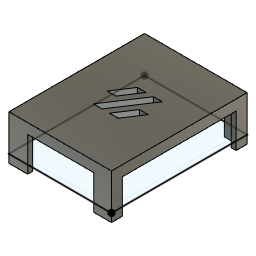
BME Box v3 (Autodesk Fusion 360 design; units mm, degrees)
Autodesk Fusion 360 part; units mm, degrees
sketch "Sketch1" plane through (0, 0, 0) normal (0, 0, 1) x (1, 0, 0)
  line L0 (0, 0) -> (31, 0)
  line L1 (31, 0) -> (31, 41)
  line L2 (31, 41) -> (0, 41)
  line L3 (0, 41) -> (0, 0)
  line L4 (1.5, 39.5) -> (29.5, 39.5)
  line L5 (29.5, 39.5) -> (29.5, 1.5)
  line L6 (29.5, 1.5) -> (1.5, 1.5)
  line L7 (1.5, 1.5) -> (1.5, 39.5)
  line L8 (1.5, 39.5) -> (29.5, 1.5) construction
  line L9 (29.5, 39.5) -> (1.5, 1.5) construction
  circle A0 centre (15.5, 28.7333) radius 7.5
  point P0 (15.5, 20.5)
  dimension "d1" = 31
  dimension "d2" = 41
  dimension "d3" = 28
  dimension "d4" = 38
  dimension "d5" = 15
  constraint horizontal L0
  constraint vertical L1
  constraint horizontal L2
  constraint vertical L3
  constraint coincident L0.start L3.end
  constraint horizontal L4
  constraint perpendicular L4 L5
  constraint parallel L4 L6
  constraint parallel L5 L7
  constraint coincident L8 P0
  constraint coincident L9 P0
  measures "d1" distance of L0.start L0.end
  measures "d2" distance of L0.start L2.end
  measures "d3" distance of L5.end L6.end
  measures "d4" distance of L4.end L5.end
  measures "d5" diameter of A0
extrude "Extrude1" add sketch "Sketch1" along normal blind 2 contours L0 L1 L2 L3 | L4 L5 L6 L7 makes body 1
extrude "Extrude2" add sketch "Sketch1" along normal blind 4 contours L4 L5 L6 L7 bodies 1
sketch "Sketch1 (2)" plane through (0, 0, 2) normal (0, 0, 1) x (-1, 0, 0) in component "Top"
  line L0 (-1.5, -1.5) -> (-1.5, -39.5)
  line L1 (-1.5, -39.5) -> (-29.5, -39.5)
  line L2 (-29.5, -39.5) -> (-29.5, -1.5)
  line L3 (-29.5, -1.5) -> (-1.5, -1.5)
  line L4 (0, -41) -> (0, 0)
  line L5 (0, 0) -> (-31, 0)
  line L6 (-31, 0) -> (-31, -41)
  line L7 (-31, -41) -> (0, -41)
  line L8 (0, -41) -> (-31, -41)
  line L9 (-31, -41) -> (-31, 0)
  line L10 (-31, 0) -> (0, 0)
  line L11 (0, 0) -> (0, -41)
  constraint horizontal L8
  constraint vertical L9
  constraint horizontal L10
  constraint vertical L11
  constraint coincident L5.end L6.start
  constraint coincident L4.start L7.end
extrude "Extrude1'" add sketch "Sketch1 (2)" along normal blind 10 separate body contours L0 L1 L2 L3 | L4 L5 L6 L7 L8 L9 L10 L11 makes body 2 in component "Top"
shell "Shell1" thickness 1.5 removed faces 1 at (10.3333, 27.3333, 2) on bodies 2 in component "Top"
ref_plane "WorkPlane1" through (15.5, 20.5, 12) normal (0, 0, 1) x (1, 0, 0)
sketch "Sketch2" plane through (15.5, 20.5, 12) normal (0, 0, 1) x (1, 0, 0) in component "Top"
  line L0 (0.1136, 9.8824) -> (-8.6176, 4.8413)
  line L1 (-8.6176, 4.8413) -> (-8.6176, -5.2393)
  line L2 (-8.6176, -5.2393) -> (0.1136, -10.2796)
  line L3 (0.1136, -10.2796) -> (8.8449, -5.2393)
  line L4 (8.8449, -5.2393) -> (8.8449, 4.8413)
  line L5 (8.8449, 4.8413) -> (0.1136, 9.8824)
  line L6 (-2.4502, 5.2787) -> (0.1835, 5.2787)
  line L7 (0.1835, 5.2787) -> (-3.4193, -0.2014)
  line L8 (-3.4193, -0.2014) -> (-6.053, -0.2014)
  line L9 (-6.053, -0.2014) -> (-2.4502, 5.2787)
  line L10 (-4.8021, -5.6751) -> (2.4028, 5.2866)
  line L11 (2.4028, 5.2866) -> (5.0365, 5.2866)
  line L12 (5.0365, 5.2866) -> (-2.1692, -5.6751)
  line L13 (-2.1692, -5.6751) -> (-4.8021, -5.6751)
  line L14 (2.6854, -5.6751) -> (0.0517, -5.6751)
  line L15 (0.0517, -5.6751) -> (3.6538, -0.195)
  line L16 (3.6538, -0.195) -> (6.2874, -0.195)
  line L17 (6.2874, -0.195) -> (2.6854, -5.6751)
extrude "Extrude2'" cut sketch "Sketch2" against normal blind 0.5 bodies 2 in component "Top"
extrude "Extrude3" cut 3 faces at (19.7089, 18.4783, 12) (17.2567, 22.1327, 12) (13.6047, 23.952, 12) along direction (0, 0, -1) blind 2 on bodies 2 bodies 2 in component "Top"
sketch "Sketch2 (1)" plane through (0, 41, 0) normal (0, 1, 0) x (-1, 0, 0) in component "Top"
  line L0 (-31, 2) -> (0, 2)
  line L1 (0, 2) -> (0, 12)
  line L2 (0, 12) -> (-31, 12)
  line L3 (-31, 12) -> (-31, 2)
  line L4 (-28.0584, 2) -> (-2.1668, 2)
  line L5 (-2.1668, 2) -> (-2.1668, 9.9165)
  line L6 (-2.1668, 9.9165) -> (-28.0584, 9.9165)
  line L7 (-28.0584, 9.9165) -> (-28.0584, 2)
  point P0 (-15.5, 7)
  constraint horizontal L4
  constraint vertical L5
  constraint horizontal L6
  constraint vertical L7
  constraint coincident L0 L4.start
sketch "Sketch3" plane through (31, 0, 0) normal (1, 0, 0) x (0, 1, 0) in component "Top"
  line L0 (0, 2) -> (41, 2)
  line L1 (41, 2) -> (41, 12)
  line L2 (41, 12) -> (0, 12)
  line L3 (0, 12) -> (0, 2)
  line L4 (3.2975, 9.8315) -> (37.7025, 9.8315)
  line L5 (37.7025, 9.8315) -> (37.7025, 4.1685)
  line L6 (37.7025, 4.1685) -> (3.2975, 4.1685)
  line L7 (3.2975, 4.1685) -> (3.2975, 9.8315)
  line L8 (3.2975, 9.8315) -> (37.7025, 4.1685) construction
  line L9 (37.7025, 9.8315) -> (3.2975, 4.1685) construction
  point P0 (20.5, 7)
  constraint horizontal L4
  constraint perpendicular L4 L5
  constraint parallel L4 L6
  constraint parallel L5 L7
  constraint coincident L8 P0
  constraint coincident L9 P0
extrude "Extrude5" cut sketch "Sketch3" against normal blind 35 contours L4 L5 L6 L7 bodies 2 in component "Top"
extrude "Extrude6" add 1 faces at (15.5379, 37.4608, 12) along direction (0, 0, 1) blind 1 on bodies 2 bodies 2 in component "Top"
extrude "Extrude7" add 1 faces at (9.7931, 23.8062, 11.5) along direction (0, 0, 1) blind 1.5 on bodies 2 bodies 2 in component "Top"
extrude "Extrude8" cut 1 faces at (15.5612, 35.9262, 13) along direction (0, 0, 1) blind 1 on bodies 2 bodies 2 in component "Top"
extrude "Extrude9" add sketch "Sketch1 (2)" against normal blind 2.5 bodies 2 in component "Top"
sketch "Sketch4" plane through (0, 0, 0) normal (-1, 0, 0) x (0, -1, 0) in component "Top"
  line L0 (-37.7025, 4.1685) -> (-37.7025, 9.8315)
  line L1 (-37.7025, 9.8315) -> (-3.2975, 9.8315)
  line L2 (-3.2975, 9.8315) -> (-3.2975, 4.1685)
  line L3 (-3.2975, 4.1685) -> (-37.7025, 4.1685)
  line L4 (0, -0.5) -> (0, 13)
  line L5 (0, 13) -> (-41, 13)
  line L6 (-41, 13) -> (-41, -0.5)
  line L7 (-41, -0.5) -> (0, -0.5)
  line L8 (-37.7025, 9.8315) -> (-3.2975, 9.8315)
  line L9 (-3.2975, 9.8315) -> (-3.2975, -1.832)
  line L10 (-3.2975, -1.832) -> (-37.7025, -1.832)
  line L11 (-37.7025, -1.832) -> (-37.7025, 9.8315)
  constraint horizontal L8
  constraint vertical L9
  constraint horizontal L10
  constraint vertical L11
  constraint coincident L2 L9.end
  constraint coincident L0.end L1.start
extrude "Extrude10" cut sketch "Sketch4" against normal blind 45.044 contours L0 L1 L2 L3 L8 L9 L11 | L3 L7 L9 L11 | L7 L9 L10 L11 bodies 2 in component "Top"
sketch "Sketch5" plane through (0, 0, 0) normal (0, -1, 0) x (1, 0, 0) in component "Top"
  line L0 (31, -0.5) -> (31, 13)
  line L1 (31, 13) -> (0, 13)
  line L2 (0, 13) -> (0, -0.5)
  line L3 (0, -0.5) -> (31, -0.5)
  line L4 (5.6791, -0.5) -> (25.6474, -0.5)
  line L5 (25.6474, -0.5) -> (25.6474, 9.8926)
  line L6 (25.6474, 9.8926) -> (5.6791, 9.8926)
  line L7 (5.6791, 9.8926) -> (5.6791, -0.5)
  constraint horizontal L4
  constraint vertical L5
  constraint horizontal L6
  constraint vertical L7
  constraint coincident L3 L4.start
extrude "Extrude11" cut sketch "Sketch5" against normal blind 159.301 contours L3 L4 L5 L6 L7 bodies 2 in component "Top"
component "Top" placed x (1, 0, 0) y (0, 1, 0) z (0, 0, 1) at (0, 0, 0)
hidden bodies 1
